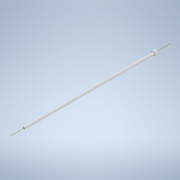
# Autodesk Inventor part: balanceRod
Saved by Autodesk Inventor 2020 (Build 240168000, 168)
## iProperties
Created: 2022-12-14
Part Number: balanceRod
Material: Generic
Document SubType Name: Modeling
Designer: Manish
Density: 1 g/cm^3
Appearance: Default
Author: Manish
Autodesk Inventor part; units mm, degrees
ref_plane "YZ Plane" through (0, 0, 0) normal (1, 0, 0) x (0, 1, 0)
ref_plane "XZ Plane" through (0, 0, 0) normal (0, 1, 0) x (-1, 0, 0)
ref_plane "XY Plane" through (0, 0, 0) normal (0, 0, 1) x (1, 0, 0)
sketch "Sketch1" plane through (0, 0, 0) normal (0, 0, 1) x (1, 0, 0)
  circle A0 centre (0, 0) radius 4
  dimension "d0" = 8
  constraints: 1 centre point, 1 coincident
  measures "d0" diameter of A0
extrude "Extrusion1" add sketch "Sketch1" against normal blind 450
sketch "Sketch3" plane through (0, 0, -450) normal (0, 0, -1) x (-1, 0, 0)
  circle A0 centre (0, 0) radius 6.6654
  constraints: 1 centre point, 1 coincident
extrude "Extrusion2" add sketch "Sketch3" against normal blind 20
body "Solid1"
